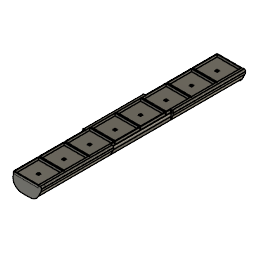
Tabla (Autodesk Fusion 360 design; units mm, degrees)
part number: 2026-06-05-10-17-05-471
Autodesk Fusion 360 part; units mm, degrees
note: some values were not read from the file. Set by a fixed rule: which sketch regions a step uses.
sketch "Sketch2" plane through (0, 0, 0) normal (0, 0, 1) x (1, 0, 0)
  line L0 (0, 0) -> (21, 0)
  line L1 (21, 0) -> (21, 21)
  line L2 (21, 21) -> (0, 21)
  line L3 (0, 21) -> (0, 0)
  line L4 (20.5, 0.5) -> (20.5, 20.5)
  line L5 (20.5, 20.5) -> (0.5, 20.5)
  line L6 (0.5, 20.5) -> (0.5, 0.5)
  line L7 (0.5, 0.5) -> (20.5, 0.5)
  line L8 (0, 21) -> (21, 21)
  line L9 (21, 21) -> (21, 21.25)
  line L10 (21, 21.25) -> (0, 21.25)
  line L11 (0, 21.25) -> (0, 21)
  dimension "d14" = 21
  dimension "d15" = 21
  dimension "d16" = -0.5
  dimension "d17" = 21
  dimension "d18" = 0.25
  constraint horizontal L0
  constraint vertical L1
  constraint horizontal L2
  constraint vertical L3
  constraint coincident L0.start L3.end
  constraint horizontal L8
  constraint vertical L9
  constraint horizontal L10
  constraint vertical L11
  measures "d14" distance of L0.start L0.end
  measures "d15" distance of L0.start L2.end
  measures "d17" distance of L2.end L1.end
  measures "d18" distance of L2.end L10.end
extrude "Extrude4" add sketch "Sketch2" along normal blind 10 contours L0 L1 L2 L3 L8 makes body 1
extrude "Extrude5" add sketch "Sketch2" along normal blind 8 contours L4 L5 L6 L7 bodies 1
extrude "Extrude8" add sketch "Sketch2" along normal blind 8 contours L2 L8 L9 L10 L11 bodies 1
extrude "Extrude6" add sketch "Sketch2" along normal blind 8 contours L2 L8 L9 L10 L11 bodies 1
sketch "Sketch3" plane through (0, 0, 8) normal (0, 0, 1) x (-1, 0, 0)
  line L0 (-0.5, -0.5) -> (-20.5, -0.5)
  line L1 (-20.5, -0.5) -> (-20.5, -20.5)
  line L2 (-20.5, -20.5) -> (-0.5, -20.5)
  line L3 (-0.5, -20.5) -> (-0.5, -0.5)
  line L4 (-0.5, -0.5) -> (-9.5, -0.5)
  line L5 (-0.5, -9.5) -> (-0.5, -0.5)
  line L6 (-9.5, -9.5) -> (-11.5, -9.5)
  line L7 (-11.5, -9.5) -> (-11.5, -11.5)
  line L8 (-11.5, -11.5) -> (-9.5, -11.5)
  line L9 (-9.5, -11.5) -> (-9.5, -9.5)
  dimension "d25" = 9
  dimension "d26" = 9
  dimension "d27" = 2
  dimension "d28" = 2
  constraint horizontal L4
  constraint vertical L5
  constraint coincident L0.start L3.end
  constraint horizontal L6
  constraint vertical L7
  constraint horizontal L8
  constraint vertical L9
  measures "d25" distance of L0.start L4.end
  measures "d26" distance of L0.start L5.start
  measures "d27" distance of L6.start L6.end
  measures "d28" distance of L6.start L8.end
extrude "Extrude7" cut sketch "Sketch3" against normal blind 1 contours L6 L7 L8 L9 bodies 1
copy_body "CopyPasteBodies1" bodies 1 makes body 2
move_body "Move1" bodies 2 to x (1, 0, 0) y (0, 1, 0) z (0, 0, 1) at (0, 21.25, 0)
combine "Combine1" operation add target body 1 tool bodies 2
copy_body "CopyPasteBodies2" bodies 1 makes body 3
move_body "Move2" bodies 3 to x (1, 0, 0) y (0, 1, 0) z (0, 0, 1) at (0, 42.5, 0)
combine "Combine2" operation add target body 1 tool bodies 3
copy_body "CopyPasteBodies3" bodies 1 makes body 4
move_body "Move3" bodies 4 to x (1, 0, 0) y (0, 1, 0) z (0, 0, 1) at (0, 85, 0)
combine "Combine3" operation add target body 1 tool bodies 4
move_body "Move4" bodies 1 to x (-1, 0, 0) y (0, 1, 0) z (0, 0, -1) at (0, 0, 0)
move_body "Move5" bodies 1 to x (1, 0, 0) y (0, 1, 0) z (0, 0, 1) at (0, 0, 10)
sketch "Sketch4" plane through (0, 0, 10) normal (0, 0, 1) x (-1, 0, 0)
  line L0 (21, -170) -> (21, 0)
  line L1 (21, 0) -> (0, 0)
  line L2 (0, 0) -> (0, -170)
  line L3 (0, -170) -> (21, -170)
  line L4 (21, 0) -> (0, 0)
  line L5 (0, 0) -> (0, -170)
  line L6 (0, -170) -> (21, -170)
  line L7 (21, -170) -> (21, 0)
  constraint horizontal L4
  constraint vertical L5
  constraint horizontal L6
  constraint vertical L7
  constraint coincident L2.end L3.start
  constraint coincident L0.end L1.start
sketch "Sketch5" plane through (0, 0, 0) normal (0, -1, 0) x (1, 0, 0)
  line L0 (0, 10) -> (-21, 10)
  line L1 (-21, 10) -> (-21, 0)
  line L2 (-21, 0) -> (0, 0)
  line L3 (0, 0) -> (0, 10)
  arc A0 (0, 10) -> (-21, 10) centre (-10.5, -12.7431) ccw
  dimension "d34" = 25.0499
  constraint coincident L0.start L3.end
  constraint coincident L0.end L1.start
  measures "d34" radius of A0
extrude "Extrude9" add sketch "Sketch5" against normal blind 170 contours L0 A0 bodies 1
fillet "Fillet1" radius 6 2 edges at (-21, 85, 10) (0, 85, 10) on bodies 1
move_body "Move6" bodies 1 to x (-1, 0, 0) y (0, 1, 0) z (0, 0, -1) at (-42, 0, 0)
move_body "Move7" bodies 1 to x (1, 0, 0) y (0, 1, 0) z (0, 0, 1) at (0, 0, 20)
sketch "Sketch6" plane through (0, 11.5, 0) normal (0, -1, 0) x (1, 0, 0)
  line L0 (-30.5, 18) -> (-32.5, 18)
  line L1 (-32.5, 18) -> (-32.5, 17)
  line L2 (-32.5, 17) -> (-30.5, 17)
  line L3 (-30.5, 17) -> (-30.5, 18)
sketch "Sketch7" plane through (0, 20.5, 0) normal (0, -1, 0) x (1, 0, 0)
  line L0 (-41.5, 18) -> (-21.5, 18)
  line L1 (-21.5, 18) -> (-21.5, 20)
  line L2 (-21.5, 20) -> (-41.5, 20)
  line L3 (-41.5, 20) -> (-41.5, 18)
sketch "Sketch8" plane through (3, 0, 0) normal (1, 0, 0) x (0, 1, 0)
  line L0 (0, 14.2323) -> (170, 14.2323)
  line L1 (170, 14.2323) -> (170, 18)
  line L2 (170, 18) -> (169.75, 18)
  line L3 (169.75, 18) -> (169.75, 20)
  line L4 (169.75, 20) -> (148.75, 20)
  line L5 (148.75, 20) -> (148.75, 18)
  line L6 (148.75, 18) -> (148.5, 18)
  line L7 (148.5, 18) -> (148.5, 20)
  line L8 (148.5, 20) -> (127.5, 20)
  line L9 (127.5, 20) -> (127.5, 18)
  line L10 (127.5, 18) -> (127.25, 18)
  line L11 (127.25, 18) -> (127.25, 20)
  line L12 (127.25, 20) -> (106.25, 20)
  line L13 (106.25, 20) -> (106.25, 18)
  line L14 (106.25, 18) -> (106, 18)
  line L15 (106, 18) -> (106, 20)
  line L16 (106, 20) -> (85, 20)
  line L17 (85, 20) -> (85, 18)
  line L18 (85, 18) -> (84.75, 18)
  line L19 (84.75, 18) -> (84.75, 20)
  line L20 (84.75, 20) -> (63.75, 20)
  line L21 (63.75, 20) -> (63.75, 18)
  line L22 (63.75, 18) -> (63.5, 18)
  line L23 (63.5, 18) -> (63.5, 20)
  line L24 (63.5, 20) -> (42.5, 20)
  line L25 (42.5, 20) -> (42.5, 18)
  line L26 (42.5, 18) -> (42.25, 18)
  line L27 (42.25, 18) -> (42.25, 20)
  line L28 (42.25, 20) -> (21.25, 20)
  line L29 (21.25, 20) -> (21.25, 18)
  line L30 (21.25, 18) -> (21, 18)
  line L31 (21, 18) -> (21, 20)
  line L32 (21, 20) -> (0, 20)
  line L33 (0, 20) -> (0, 14.2323)
sketch "Sketch9" plane through (0, 0, 0) normal (0, -1, 0) x (1, 0, 0)
  arc A0 (-18, 14.2323) -> (-13.4173, 8.4021) centre (-12, 14.2323) ccw
  arc A1 (-13.4173, 8.4021) -> (-1.5827, 8.4021) centre (-7.5, 32.7431) ccw
  arc A2 (-1.5827, 8.4021) -> (3, 14.2323) centre (-3, 14.2323) ccw
  line L0 (3, 14.2323) -> (3, 20)
  line L1 (3, 20) -> (-18, 20)
  line L2 (-18, 20) -> (-18, 14.2323)
  line L3 (3, 19.4) -> (3, 19.8)
  arc A3 (3.2, 19.6) -> (3, 19.8) centre (3, 19.6) ccw
  line L4 (3.2, 19.6) -> (3.2, 19.5)
  line L5 (3.2, 19.5) -> (3, 19.109)
  point P0 (3.2, 19.8)
  dimension "d42" = 0.2
  dimension "d43" = 0.4
  dimension "d44" = 0.2
  constraint vertical L3
  constraint coincident L0 L3.end
  constraint coincident L3.end A3.end
  constraint parallel L3 L4
  constraint coincident L0 L5.end
  measures "d42" distance of L3.end P0
  measures "d43" distance of L3.end L3.start
  measures "d44" radius of A3
move_body "Move13" bodies 1 to x (1, 0, 0) y (0, 1, 0) z (0, 0, 1) at (31.5, 0, -7.6932)
sketch "Sketch11" plane through (0, 0, 0) normal (0, -1, 0) x (1, 0, 0)
  arc A0 (-10.5, 6.5391) -> (-5.9173, 0.7089) centre (-4.5, 6.5391) ccw
  arc A1 (-5.9173, 0.7089) -> (5.9173, 0.7089) centre (0, 25.0499) ccw
  arc A2 (5.9173, 0.7089) -> (10.5, 6.5391) centre (4.5, 6.5391) ccw
  line L0 (10.5, 6.5391) -> (10.5, 12.3068)
  line L1 (10.5, 12.3068) -> (-10.5, 12.3068)
  line L2 (-10.5, 12.3068) -> (-10.5, 6.5391)
  line L3 (10.5, 12.3068) -> (11.8, 12.3068)
  line L4 (13, 11.1068) -> (13, 10.9591)
  line L5 (13, 9.8068) -> (10.5, 9.8068)
  line L6 (10.5, 9.8068) -> (10.5, 12.3068)
  line L7 (12.4957, 8.7708) -> (10.4161, 4.4986)
  line L8 (0, 0) -> (3.223, 0)
  arc A3 (13, 11.1068) -> (11.8, 12.3068) centre (11.8, 11.1068) ccw
  arc A4 (12.4957, 8.7708) -> (13, 10.9591) centre (8, 10.9591) ccw
  arc A5 (3.223, 0) -> (10.4161, 4.4986) centre (3.223, 8) ccw
  circle A6 centre (11.8, 11.1068) radius 0.875
  circle A7 centre (-11.8, 11.1068) radius 0.875
  arc A8 (-13, 10.9591) -> (-12.4957, 8.7708) centre (-8, 10.9591) ccw
  line L9 (-10.5, 12.3068) -> (-11.8, 12.3068)
  arc A9 (-11.8, 12.3068) -> (-13, 11.1068) centre (-11.8, 11.1068) ccw
  line L10 (-12.4957, 8.7708) -> (-10.4161, 4.4986)
  line L11 (-13, 11.1068) -> (-13, 10.9591)
  line L12 (-13, 9.8068) -> (-10.5, 9.8068)
  arc A10 (-10.4161, 4.4986) -> (-3.223, 0) centre (-3.223, 8) ccw
  line L13 (-3.223, 0) -> (0, 0)
  line L14 (0, 0) -> (3.223, 0)
  arc A11 (3.223, 0) -> (10.4161, 4.4986) centre (3.223, 8) ccw
  line L15 (12.4957, 8.7708) -> (10.4161, 4.4986)
  arc A12 (13, 11.1068) -> (11.8, 12.3068) centre (11.8, 11.1068) ccw
  line L16 (10.5, 12.3068) -> (11.8, 12.3068)
  circle A13 centre (11.8, 11.1068) radius 0.875
  line L17 (13, 11.1068) -> (13, 10.9591)
  arc A14 (12.4957, 8.7708) -> (13, 10.9591) centre (8, 10.9591) ccw
  line L18 (10.4161, 4.4986) -> (10.907, 7.4657)
  line L19 (10.5, 9.8068) -> (10.4144, 9.8073)
  line L20 (0, 0) -> (0, 14)
  line L21 (10.2599, 10.1289) -> (10.5, 9.8068)
  arc A15 (10.907, 7.4657) -> (10.2599, 10.1289) centre (7.4539, 8.0369) ccw
  arc A16 (-10.2599, 10.1289) -> (-10.907, 7.4657) centre (-7.4539, 8.0369) ccw
  line L22 (-10.4161, 4.4986) -> (-10.907, 7.4657)
  point P0 (13, 12.3068)
  point P1 (-13, 12.3068)
  dimension "d50" = 2.5
  dimension "d51" = 2.5
  dimension "d52" = 1.2
  dimension "d53" = 5
  dimension "d54" = 8
  dimension "d55" = 1.75
  dimension "d56" = 64.044
  dimension "d60" = 115.956
  dimension "d67" = 1.2
  dimension "d68" = 5
  dimension "d69" = 8
  dimension "d70" = 1.75
  dimension "d71" = 115.956
  dimension "d73" = 16.562
  dimension "d76" = 9.5014
  dimension "d93" = 3.5
  constraint horizontal L3
  constraint vertical L4
  constraint horizontal L5
  constraint vertical L6
  constraint coincident L0.end L1.start
  constraint coincident L8.start L13.end
  constraint coincident P0 L3
  constraint coincident P0 L4
  constraint tangent L3 A3
  constraint tangent L4 A3
  constraint coincident L5.start L4
  constraint coincident L5.start L7
  constraint tangent L4 A4
  constraint tangent L7 A4
  constraint tangent L8 A5
  constraint tangent L7 A5
  constraint concentric A3 A6
  constraint tangent A1 L13
  constraint vertical A0.start L12.end
  constraint tangent A8 L11
  constraint tangent A8 L10
  constraint tangent A9 L11
  constraint tangent L9 A9
  constraint concentric A7 A9
  constraint vertical L12.start A8.start
  constraint vertical L12.start A9.end
  constraint equal A4 A8
  constraint equal A3 A9
  constraint equal L5 L12
  constraint vertical L12.start P1
  constraint tangent L10 A10
  constraint tangent A10 L13
  constraint tangent A1 L8
  constraint equal A5 A10
  constraint equal L4 L11
  constraint perpendicular L2 L9
  constraint equal L3 L9
  constraint equal A6 A7
  constraint horizontal L1.end P1
  constraint collinear L3 L9
  constraint equal L8 L13
  constraint equal L7 L10
  constraint horizontal L16
  constraint vertical L17
  constraint tangent A12 L16
  constraint tangent A12 L17
  constraint tangent L17 A14
  constraint tangent L15 A14
  constraint tangent L14 A11
  constraint tangent A11 L15
  constraint concentric A12 A13
  constraint tangent L8 A11
  constraint tangent L7 A11
  constraint tangent L3 A12
  constraint tangent L7 A14
  constraint tangent L4 A14
  constraint perpendicular L1 L20
  constraint symmetric L7.end L20 L10.end
  constraint tangent L21 A15
  constraint tangent L18 A15
  constraint symmetric L20 L21.start A16.start
  constraint symmetric L20 L18.end A16.end
  constraint symmetric L20 A15 A16
  measures "d50" distance of L0.end P0
  measures "d51" distance of L0.end L5.end
  measures "d52" radius of A3
  measures "d53" radius of A4
  measures "d54" radius of A5
  measures "d55" diameter of A6
  measures "d56" angle of L10 L12
  measures "d60" angle of L7 L8
  measures "d67" radius of A12
  measures "d68" radius of A14
  measures "d69" radius of A11
  measures "d70" diameter of A13
  measures "d71" angle of L14 L15
  measures "d73" angle of L7 L18
  measures "d76" vertical distance of L10.end L20.end
  measures "d93" radius of A15
extrude "Extrude13" add sketch "Sketch11" against normal blind 170 contours A1 A2 L0 L8 A5 L14 A11 L18 A15 | L0 L5 L7 A4 L15 A14 L18 A15 | L0 L3 L4 L5 L6 A3 A4 A12 L16 L17 A14 | A6 A13 bodies 1
extrude "Extrude14" cut sketch "Sketch11" against normal blind 110 contours L0 L5 L7 A4 L15 A14 L18 A15 | L0 L3 L4 L5 L6 A3 A4 A12 L16 L17 A14 bodies 1
extrude "Extrude15" add sketch "Sketch11" against normal blind 60 contours A1 A2 L0 L8 A5 L14 A11 L18 A15 | L0 L5 L7 A4 L15 A14 L18 A15 | L0 L3 L4 L5 L6 A3 A4 A12 L16 L17 A14 bodies 1
delete_face "DeleteFace1" 1 faces at (12.6707, 76.6667, 11.0197) on bodies 1
extrude "Extrude16" cut sketch "Sketch11" against normal blind 170 contours A6 A13 bodies 1
extrude "Extrude21" add sketch "Sketch11" against normal blind 170 contours A0 A1 L2 A10 L13 A16 L22 bodies 1
extrude "Extrude22" add sketch "Sketch11" against normal blind 110 contours L2 A8 L10 L12 A16 L22 | L2 A8 L9 A9 L11 L12 bodies 1
extrude "Extrude23" cut sketch "Sketch11" against normal blind 60 contours L2 A8 L10 L12 A16 L22 | L2 A8 L9 A9 L11 L12 bodies 1
extrude "Extrude24" add sketch "Sketch11" against normal blind 3 contours A6 A13 bodies 1
